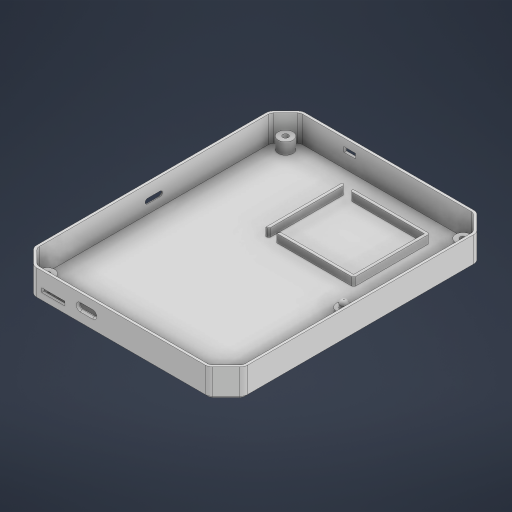
# Autodesk Inventor part: keypad_layout
Saved by Autodesk Inventor 2024 (Build 280153000, 153)
## iProperties
Created: 2023-11-21
Part Number: keypad_layout
Material: Generic
Document SubType Name: Modeling
Designer: minekuba
Density: 1 g/cm^3
Appearance: Default
Author: minekuba
Autodesk Inventor part; units mm, degrees
ref_plane "YZ Plane" through (0, 0, 0) normal (1, 0, 0) x (0, 1, 0)
ref_plane "XZ Plane" through (0, 0, 0) normal (0, 1, 0) x (-1, 0, 0)
ref_plane "XY Plane" through (0, 0, 0) normal (0, 0, 1) x (1, 0, 0)
sketch "Sketch1" plane through (0, 0, 0) normal (0, 1, 0) x (-1, 0, 0)
  line L0 (51.2574, 80) -> (-51.2574, 80)
  line L1 (-62.5, 68.7574) -> (-62.5, -68.7574)
  line L2 (-51.2574, -80) -> (51.2574, -80)
  line L3 (62.5, 80) -> (-62.5, -80) construction
  line L4 (-62.5, 80) -> (62.5, -80) construction
  line L5 (60.6213, 71.8787) -> (53.3787, 79.1213)
  line L6 (60.6213, -71.8787) -> (53.3787, -79.1213)
  line L7 (-53.3787, -79.1213) -> (-61.6213, -70.8787)
  line L8 (-53.3787, 79.1213) -> (-61.6213, 70.8787)
  arc A0 (61.5, 69.7574) -> (60.6213, 71.8787) centre (58.5, 69.7574) ccw
  arc A1 (53.3787, 79.1213) -> (51.2574, 80) centre (51.2574, 77) ccw
  arc A2 (-51.2574, 80) -> (-53.3787, 79.1213) centre (-51.2574, 77) ccw
  arc A3 (-61.6213, 70.8787) -> (-62.5, 68.7574) centre (-59.5, 68.7574) ccw
  arc A4 (-62.5, -68.7574) -> (-61.6213, -70.8787) centre (-59.5, -68.7574) ccw
  arc A5 (-53.3787, -79.1213) -> (-51.2574, -80) centre (-51.2574, -77) ccw
  arc A6 (60.6213, -71.8787) -> (61.5, -69.7574) centre (58.5, -69.7574) ccw
  arc A7 (51.2574, -80) -> (53.3787, -79.1213) centre (51.2574, -77) ccw
  line L9 (60.5, 42) -> (56.5, 42)
  line L10 (55.5, 41) -> (55.5, 23)
  line L11 (56.5, 22) -> (60.5, 22)
  line L12 (61.5, -69.7574) -> (61.5, 21)
  line L13 (61.5, 43) -> (61.5, 69.7574)
  arc A8 (60.5, 42) -> (61.5, 43) centre (60.5, 43) ccw
  arc A9 (56.5, 42) -> (55.5, 41) centre (56.5, 41) ccw
  arc A10 (55.5, 23) -> (56.5, 22) centre (56.5, 23) ccw
  arc A11 (61.5, 21) -> (60.5, 22) centre (60.5, 21) ccw
  circle A12 centre (54, 72.5) radius 1.65
  line L14 (67, 0) -> (-74, 0) construction
  line L15 (54, 72.5) -> (57, 75.5) construction
  circle A13 centre (54, -72.5) radius 1.65
  line L16 (0, 82) -> (0, -121) construction
  circle A14 centre (-54, 72.5) radius 1.65
  circle A15 centre (-54, -72.5) radius 1.65
  circle A16 centre (-54, 0) radius 1.65
  point P0 (0, 0)
  point P1 (62.5, 70)
  point P2 (52.5, 80)
  point P3 (62.5, -70)
  point P4 (52.5, -80)
  point P5 (-52.5, -80)
  point P6 (-62.5, -70)
  point P7 (-52.5, 80)
  point P8 (-62.5, 70)
  point P9 (55.5, 22)
  point P10 (61.5, 22)
  point P11 (58.5, 42)
  point P12 (58.5, 22)
  dimension "d0" = 125
  dimension "d1" = 160
  dimension "d2" = 10
  dimension "d3" = 10
  dimension "d4" = 10
  dimension "d5" = 10
  dimension "d6" = 10
  dimension "d7" = 10
  dimension "d8" = 10
  dimension "d9" = 10
  dimension "d10" = 3
  dimension "d11" = 38
  dimension "d12" = 102
  dimension "d13" = 6
  dimension "d14" = 1
  dimension "d15" = 3.3
  dimension "d17" = 3
  constraints: 34 end point, 26 tangent, 25 point on line, 24 point on circle, 17 centre point, 11 equal radius, 5 midpoint, 4 parallel, 3 horizontal, 3 perpendicular, 3 symmetric about line, 1 line through centre, 1 vertical, 3 other
  measures "d0" distance of L4.end L3.end
  measures "d1" distance of L3.end L4.start
  measures "d2" distance of point (62.5, 70) L3.start
  measures "d3" distance of point (52.5, 80) L3.start
  measures "d4" distance of point (62.5, -70) L4.end
  measures "d5" distance of point (52.5, -80) L4.end
  measures "d6" distance of point (-52.5, -80) L3.end
  measures "d7" distance of point (-62.5, -70) L3.end
  measures "d8" distance of point (-52.5, 80) L4.start
  measures "d9" distance of point (-62.5, 70) L4.start
  measures "d10" radius of A0
  measures "d11" distance from line of L0 point (58.5, 42)
  measures "d12" distance from line of L2 point (58.5, 22)
  measures "d13" distance of point (55.5, 22) point (61.5, 22)
  measures "d14" radius of A8
  measures "d15" diameter of A12
  measures "d17" horizontal distance of L15.start L15.end
sketch "Sketch2" plane through (0, 0, 0) normal (0, 1, 0) x (-1, 0, 0)
  line L0 (60.6213, -71.8787) -> (53.3787, -79.1213) construction
  arc A0 (51.2574, -80) -> (53.3787, -79.1213) centre (51.2574, -77) ccw construction
  arc A1 (60.6213, -71.8787) -> (61.5, -69.7574) centre (58.5, -69.7574) ccw construction
  line L1 (61.5, -69.7574) -> (61.5, 21) construction
  arc A2 (61.5, 21) -> (60.5, 22) centre (60.5, 21) ccw construction
  line L2 (56.5, 22) -> (60.5, 22) construction
  arc A3 (55.5, 23) -> (56.5, 22) centre (56.5, 23) ccw construction
  line L3 (55.5, 41) -> (55.5, 23) construction
  arc A4 (56.5, 42) -> (55.5, 41) centre (56.5, 41) ccw construction
  arc A5 (60.5, 42) -> (61.5, 43) centre (60.5, 43) ccw construction
  line L4 (61.5, 43) -> (61.5, 69.7574) construction
  arc A6 (61.5, 69.7574) -> (60.6213, 71.8787) centre (58.5, 69.7574) ccw construction
  line L5 (60.6213, 71.8787) -> (53.3787, 79.1213) construction
  arc A7 (53.3787, 79.1213) -> (51.2574, 80) centre (51.2574, 77) ccw construction
  line L6 (51.2574, 80) -> (-51.2574, 80) construction
  arc A8 (-51.2574, 80) -> (-53.3787, 79.1213) centre (-51.2574, 77) ccw construction
  line L7 (-53.3787, 79.1213) -> (-61.6213, 70.8787) construction
  arc A9 (-61.6213, 70.8787) -> (-62.5, 68.7574) centre (-59.5, 68.7574) ccw construction
  line L8 (-62.5, 68.7574) -> (-62.5, -68.7574) construction
  arc A10 (-62.5, -68.7574) -> (-61.6213, -70.8787) centre (-59.5, -68.7574) ccw construction
  line L9 (-53.3787, -79.1213) -> (-61.6213, -70.8787) construction
  arc A11 (-53.3787, -79.1213) -> (-51.2574, -80) centre (-51.2574, -77) ccw construction
  line L10 (-51.2574, -80) -> (51.2574, -80) construction
  line L11 (60.5, 42) -> (56.5, 42) construction
  line L12 (53.5201, 79.2627) -> (60.7627, 72.0201)
  arc A12 (61.7, 69.7574) -> (60.7627, 72.0201) centre (58.5, 69.7574) ccw
  line L13 (61.7, 69.7574) -> (61.7, 43)
  line L14 (61.7, 21) -> (61.7, -69.7574)
  arc A13 (60.7627, -72.0201) -> (61.7, -69.7574) centre (58.5, -69.7574) ccw
  line L15 (60.7627, -72.0201) -> (53.5201, -79.2627)
  arc A14 (51.2574, -80.2) -> (53.5201, -79.2627) centre (51.2574, -77) ccw
  line L16 (51.2574, -80.2) -> (-51.2574, -80.2)
  arc A15 (-53.5201, -79.2627) -> (-51.2574, -80.2) centre (-51.2574, -77) ccw
  line L17 (-53.5201, -79.2627) -> (-61.7627, -71.0201)
  arc A16 (-62.7, -68.7574) -> (-61.7627, -71.0201) centre (-59.5, -68.7574) ccw
  line L18 (-62.7, -68.7574) -> (-62.7, 68.7574)
  arc A17 (-61.7627, 71.0201) -> (-62.7, 68.7574) centre (-59.5, 68.7574) ccw
  line L19 (-61.7627, 71.0201) -> (-53.5201, 79.2627)
  arc A18 (-51.2574, 80.2) -> (-53.5201, 79.2627) centre (-51.2574, 77) ccw
  line L20 (-51.2574, 80.2) -> (51.2574, 80.2)
  arc A19 (53.5201, 79.2627) -> (51.2574, 80.2) centre (51.2574, 77) ccw
  line L21 (61.7, 43) -> (61.7, 21)
  line L22 (63.2, 43) -> (63.2, 69.7574)
  arc A20 (63.2, 69.7574) -> (61.8234, 73.0808) centre (58.5, 69.7574) ccw
  line L23 (61.8234, 73.0808) -> (54.5808, 80.3234)
  arc A21 (54.5808, 80.3234) -> (51.2574, 81.7) centre (51.2574, 77) ccw
  line L24 (51.2574, 81.7) -> (-51.2574, 81.7)
  arc A22 (-51.2574, 81.7) -> (-54.5808, 80.3234) centre (-51.2574, 77) ccw
  line L25 (-54.5808, 80.3234) -> (-62.8234, 72.0808)
  arc A23 (-62.8234, 72.0808) -> (-64.2, 68.7574) centre (-59.5, 68.7574) ccw
  line L26 (-64.2, 68.7574) -> (-64.2, -68.7574)
  arc A24 (-64.2, -68.7574) -> (-62.8234, -72.0808) centre (-59.5, -68.7574) ccw
  line L27 (-62.8234, -72.0808) -> (-54.5808, -80.3234)
  arc A25 (-54.5808, -80.3234) -> (-51.2574, -81.7) centre (-51.2574, -77) ccw
  line L28 (-51.2574, -81.7) -> (51.2574, -81.7)
  arc A26 (51.2574, -81.7) -> (54.5808, -80.3234) centre (51.2574, -77) ccw
  line L29 (54.5808, -80.3234) -> (61.8234, -73.0808)
  arc A27 (61.8234, -73.0808) -> (63.2, -69.7574) centre (58.5, -69.7574) ccw
  line L30 (63.2, -69.7574) -> (63.2, 21)
  line L31 (63.2, 21) -> (63.2, 43)
  point P0 (0, 0)
  dimension "d18" = 0.2
  dimension "d19" = 1.5
  constraints: 40 end point, 32 point on circle, 16 centre point, 1 vertical, 32 other
  measures "d18" distance between parallel lines of L5 L12
  measures "d19" distance between parallel lines of L13 L22
extrude "Extrusion1" add sketch "Sketch2" along normal blind 1.5 contours L12 A12 L13 L21 L14 A13 L15 A14 L16 A15 L17 A16 L18 A17 L19 A18 L20 A19 | L31 L30 A27 L29 A26 L28 A25 L27 A24 L26 A23 L25 A22 L24 A21 L23 A20 L22
sketch "Sketch4" plane through (0, 1.5, 0) normal (0, 1, 0) x (1, 0, 0)
  arc A0 (-63.2, -69.7574) -> (-61.8234, -73.0808) centre (-58.5, -69.7574) ccw projected
  line L0 (-61.8234, -73.0808) -> (-54.5808, -80.3234) projected
  arc A1 (-54.5808, -80.3234) -> (-51.2574, -81.7) centre (-51.2574, -77) ccw projected
  line L1 (-51.2574, -81.7) -> (51.2574, -81.7) projected
  arc A2 (51.2574, -81.7) -> (54.5808, -80.3234) centre (51.2574, -77) ccw projected
  line L2 (54.5808, -80.3234) -> (62.8234, -72.0808) projected
  arc A3 (62.8234, -72.0808) -> (64.2, -68.7574) centre (59.5, -68.7574) ccw projected
  line L3 (64.2, -68.7574) -> (64.2, 68.7574) projected
  arc A4 (64.2, 68.7574) -> (62.8234, 72.0808) centre (59.5, 68.7574) ccw projected
  line L4 (62.8234, 72.0808) -> (54.5808, 80.3234) projected
  arc A5 (54.5808, 80.3234) -> (51.2574, 81.7) centre (51.2574, 77) ccw projected
  line L5 (51.2574, 81.7) -> (-51.2574, 81.7) projected
  arc A6 (-51.2574, 81.7) -> (-54.5808, 80.3234) centre (-51.2574, 77) ccw projected
  line L6 (-54.5808, 80.3234) -> (-61.8234, 73.0808) projected
  arc A7 (-61.8234, 73.0808) -> (-63.2, 69.7574) centre (-58.5, 69.7574) ccw projected
  line L7 (-63.2, 69.7574) -> (-63.2, -69.7574) projected
  line L8 (51.2574, -80.2) -> (-51.2574, -80.2)
  arc A8 (-53.5201, -79.2627) -> (-51.2574, -80.2) centre (-51.2574, -77) ccw
  line L9 (-53.5201, -79.2627) -> (-60.7627, -72.0201)
  arc A9 (-61.7, -69.7574) -> (-60.7627, -72.0201) centre (-58.5, -69.7574) ccw
  line L10 (-61.7, -69.7574) -> (-61.7, 69.7574)
  arc A10 (-60.7627, 72.0201) -> (-61.7, 69.7574) centre (-58.5, 69.7574) ccw
  line L11 (-60.7627, 72.0201) -> (-53.5201, 79.2627)
  arc A11 (-51.2574, 80.2) -> (-53.5201, 79.2627) centre (-51.2574, 77) ccw
  line L12 (-51.2574, 80.2) -> (51.2574, 80.2)
  arc A12 (53.5201, 79.2627) -> (51.2574, 80.2) centre (51.2574, 77) ccw
  line L13 (53.5201, 79.2627) -> (61.7627, 71.0201)
  arc A13 (62.7, 68.7574) -> (61.7627, 71.0201) centre (59.5, 68.7574) ccw
  line L14 (62.7, 68.7574) -> (62.7, -68.7574)
  arc A14 (61.7627, -71.0201) -> (62.7, -68.7574) centre (59.5, -68.7574) ccw
  line L15 (61.7627, -71.0201) -> (53.5201, -79.2627)
  arc A15 (51.2574, -80.2) -> (53.5201, -79.2627) centre (51.2574, -77) ccw
  point P0 (0, 0)
  dimension "d22" = 1.5
  constraints: 16 end point, 16 point on circle, 8 centre point, 15 other
  measures "d22" distance between parallel lines of L1 L8
extrude "Extrusion2" add sketch "Sketch4" along normal blind 16
sketch "Sketch5" plane through (0, 1.5, 0) normal (0, 1, 0) x (1, 0, 0)
  circle A0 centre (-54, -72.5) radius 1.65 projected
  circle A1 centre (-54, 72.5) radius 1.65 projected
  circle A2 centre (54, 72.5) radius 1.65 projected
  circle A3 centre (54, 0) radius 1.65 projected
  circle A4 centre (54, -72.5) radius 1.65 projected
  circle A5 centre (-54, -72.5) radius 4.4426
  line L0 (-53.5201, -79.2627) -> (-60.7627, -72.0201) projected
  circle A6 centre (-54, 72.5) radius 4.4426
  line L1 (-60.7627, 72.0201) -> (-53.5201, 79.2627) projected
  circle A7 centre (54, 72.5) radius 4.4426
  line L2 (61.7627, 71.0201) -> (53.5201, 79.2627) projected
  circle A8 centre (54, 0) radius 4.4425
  circle A9 centre (54, -72.5) radius 4.4426
  line L3 (61.7627, -71.0201) -> (53.5201, -79.2627) projected
  point P0 (0, 0)
  dimension "d25" = 8.885
  constraints: 5 centre point, 5 coincident, 4 tangent
  measures "d25" diameter of A8
extrude "Extrusion3" add sketch "Sketch5" along normal blind 7 contours A3 | A5 | A6 | A7 | A8 | A9
sketch "Sketch6" plane through (51.2574, 0, -81.7) normal (0, 0, -1) x (-1, 0, 0)
  line L0 (114.4574, 0) -> (114.4574, 17.5) projected
  line L1 (0, 0) -> (102.5147, 0) projected
  line L2 (77.4574, 13) -> (70.4574, 13)
  line L3 (70.4574, 13) -> (70.4574, 10)
  line L4 (70.4574, 10) -> (77.4574, 10)
  line L5 (77.4574, 10) -> (77.4574, 13)
  point P0 (51.2574, 0)
  point P1 (77.4574, 11.5)
  dimension "d28" = 10
  dimension "d29" = 37
  dimension "d30" = 7
  dimension "d31" = 3
  constraints: 8 end point, 2 parallel, 1 horizontal, 1 midpoint, 1 perpendicular
  measures "d28" distance between parallel lines of L1 L4
  measures "d29" distance from line of L0 point (77.457, 11.5)
  measures "d30" distance of L2.start L2.end
  measures "d31" distance of L2.end L3.end
extrude "Extrusion4" cut sketch "Sketch6" against normal blind 5
sketch "Sketch7" plane through (0, 1.5, 0) normal (0, 1, 0) x (1, 0, 0)
  line L0 (-7.3, 22.2) -> (37.7, 22.2)
  line L1 (37.7, 22.2) -> (37.7, 65.2)
  line L2 (37.7, 65.2) -> (-7.3, 65.2)
  line L3 (-12.3, 65.2) -> (-12.3, 22.2)
  line L4 (-51.2574, 80.2) -> (51.2574, 80.2) projected
  line L5 (62.7, 68.7574) -> (62.7, -68.7574) projected
  line L6 (39.4, 20.5) -> (39.4, 66.9)
  line L7 (-14, 66.9) -> (-14, 20.5)
  line L8 (-12.3, 22.2) -> (-12.3, 20.5)
  line L9 (-7.3, 20.5) -> (-7.3, 22.2)
  line L10 (-14, 20.5) -> (-12.3, 20.5)
  line L11 (-7.3, 20.5) -> (39.4, 20.5)
  line L12 (-12.3, 65.2) -> (-12.3, 66.9)
  line L13 (-7.3, 65.2) -> (-7.3, 66.9)
  line L14 (39.4, 66.9) -> (-7.3, 66.9)
  line L15 (-12.3, 66.9) -> (-14, 66.9)
  point P0 (0, 0)
  point P1 (-7.3, 66.05)
  dimension "d34" = 50
  dimension "d35" = 43
  dimension "d36" = 15
  dimension "d37" = 25
  dimension "d40" = 5
  dimension "d41" = 5
  constraints: 28 end point, 10 perpendicular, 7 parallel, 1 horizontal, 1 midpoint
  measures "d34" distance of L3.start L1.end
  measures "d35" distance of L1.end L0.end
  measures "d36" distance between parallel lines of L4 L2
  measures "d37" distance between parallel lines of L5 L1
  measures "d40" distance between parallel lines of L9 L8
  measures "d41" distance from line of point (-7.3, 66.05) L12
extrude "Extrusion5" add sketch "Sketch7" along normal blind 5
sketch "Sketch8" plane through (-14, 1.5, -20.5) normal (0, 0, 1) x (1, 0, 0)
  point P0 (14, -1.5)
chamfer "Chamfer1" distance 2 angle 45 16 edges at (0, 0, -81.7) (-53.056, 0, -81.3422) (-58.2021, 0, -76.7021) (-62.8422, 0, -71.556) (-63.2, 0, 0) (-62.8422, 0, 71.556) (-58.2021, 0, 76.7021) (-53.056, 0, 81.3422) (0, 0, 81.7) (53.056, 0, 81.3422) (58.7021, 0, 76.2021) (63.8422, 0, 70.556) (64.2, 0, 0) (63.8422, 0, -70.556) (58.7021, 0, -76.2021) (53.056, 0, -81.3422)
chamfer "Chamfer2" distance 1 angle 45 6 edges at (39.4, 4, -20.5) (39.4, 4, -66.9) (-12.3, 4, -66.9) (-12.3, 4, -20.5) (-7.3, 4, -65.2) (-7.3, 4, -22.2)
sketch "Sketch10" plane through (54, 8.5, 0) normal (0, 1, 0) x (1, 0, 0)
  circle A0 centre (0, 0) radius 4.4425 projected
  circle A1 centre (0, 0) radius 2.2361
  point P0 (-54, 0)
  constraints: 1 centre point, 1 coincident
extrude "Extrusion6" add sketch "Sketch10" along normal blind 4 contours A1
fillet "Fillet1" radius 2 1 edges at (51.7639, 12.5, 0)
sketch "Sketch11" plane through (-63.2, 17.5, -69.7574) normal (-1, 0, 0) x (0, 0, 1)
  line L0 (139.5147, -15.5) -> (0, -15.5) projected
  line L1 (139.5147, -15.5) -> (139.5147, 0) projected
  line L2 (0, 0) -> (139.5147, 0) projected
  line L3 (0, -15.5) -> (0, 0) projected
  line L4 (0, -17.5) -> (139.5147, -17.5) projected
  line L5 (66.0074, -9) -> (73.5074, -9) construction
  line L6 (66.0074, -10.5) -> (73.5074, -10.5)
  line L7 (73.5074, -7.5) -> (66.0074, -7.5)
  arc A0 (66.0074, -7.5) -> (66.0074, -10.5) centre (66.0074, -9) ccw
  arc A1 (73.5074, -10.5) -> (73.5074, -7.5) centre (73.5074, -9) ccw
  point P0 (69.7574, -17.5)
  point P1 (69.7574, -9)
  point P2 (69.7574, -17.5)
  dimension "d51" = 8.5
  dimension "d52" = 1.5
  dimension "d53" = 7.5
  constraints: 8 end point, 4 point on circle, 4 tangent, 2 centre point, 2 midpoint, 2 parallel
  measures "d51" distance of point (69.757, -17.5) point (69.757, -9)
  measures "d52" radius of A1
  measures "d53" distance of L5.start L5.end
extrude "Extrusion7" cut sketch "Sketch11" against normal blind 4 contours A0 L7 A1 L6
chamfer "Chamfer3" distance 1 angle 45 4 edges at (-63.2, 10, 0) (-63.2, 8.5, 5.25) (-63.2, 7, 0) (-63.2, 8.5, -5.25)
sketch "Sketch12" plane through (-51.2574, 17.5, 81.7) normal (0, 0, 1) x (1, 0, 0)
  line L0 (0, -17.5) -> (102.5147, -17.5) projected
  line L1 (-11.9426, -15.5) -> (-11.9426, 0) projected
  line L2 (3.0574, -9) -> (17.0574, -9)
  line L3 (17.0574, -9) -> (17.0574, -11.5)
  line L4 (17.0574, -11.5) -> (3.0574, -11.5)
  line L5 (3.0574, -11.5) -> (3.0574, -9)
  point P0 (51.2574, -17.5)
  dimension "d59" = 15
  dimension "d61" = 8.5
  dimension "d62" = 14
  dimension "d63" = 2.5
  constraints: 8 end point, 2 parallel, 1 horizontal, 1 perpendicular
  measures "d59" distance between parallel lines of L1 L5
  measures "d61" distance between parallel lines of L0 L2
  measures "d62" distance of L2.start L2.end
  measures "d63" distance of L2.end L3.end
extrude "Extrusion8" cut sketch "Sketch12" against normal blind 4
sketch "Sketch14" plane through (-51.2574, 17.5, 81.7) normal (0, 0, 1) x (1, 0, 0)
  line L0 (-11.9426, -15.5) -> (-11.9426, 0) projected
  line L1 (0, -17.5) -> (102.5147, -17.5) projected
  line L2 (26.5574, -7.5) -> (34.0574, -7.5) construction
  line L3 (26.5574, -6) -> (34.0574, -6)
  line L4 (34.0574, -9) -> (26.5574, -9)
  arc A0 (26.5574, -6) -> (26.5574, -9) centre (26.5574, -7.5) ccw
  arc A1 (34.0574, -9) -> (34.0574, -6) centre (34.0574, -7.5) ccw
  point P0 (51.2574, -17.5)
  point P1 (30.3074, -7.5)
  point P2 (25.0574, -7.5)
  dimension "d66" = 37
  dimension "d67" = 8.5
  dimension "d68" = 1.5
  dimension "d69" = 7.5
  constraints: 8 end point, 5 point on circle, 4 tangent, 2 centre point, 1 horizontal, 1 midpoint, 1 parallel
  measures "d66" distance from line of point (25.057, -7.5) L0
  measures "d67" distance between parallel lines of L1 L4
  measures "d68" radius of A1
  measures "d69" distance of L2.start L2.end
extrude "Extrusion9" cut sketch "Sketch14" against normal blind 4
chamfer "Chamfer4" distance 1 angle 45 4 edges at (-20.95, 11.5, 81.7) (-15.7, 10, 81.7) (-20.95, 8.5, 81.7) (-26.2, 10, 81.7)
equation "\"d3\" = d2"
equation "\"d4\" = d2"
equation "\"d5\" = d4"
equation "\"d6\" = d2"
equation "\"d7\" = d6"
equation "\"d8\" = d2"
equation "\"d9\" = d8"
body "Solid1"
